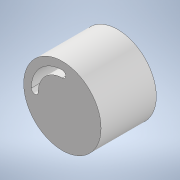
# Autodesk Inventor part: HandleGear2
Saved by Autodesk Inventor 2021 (Build 250183000, 183)
## iProperties
Created: 2021-03-29
Part Number: HandleGear2
Material: Generic
Document SubType Name: Modeling
Designer: ben
Density: 1 g/cm^3
Appearance: Default
Author: ben
Autodesk Inventor part; units mm, degrees
ref_plane "YZ Plane" through (0, 0, 0) normal (1, 0, 0) x (0, 1, 0)
ref_plane "XZ Plane" through (0, 0, 0) normal (0, 1, 0) x (-1, 0, 0)
ref_plane "XY Plane" through (0, 0, 0) normal (0, 0, 1) x (1, 0, 0)
sketch "Sketch1" plane through (0, 0, 0) normal (0, 0, 1) x (1, 0, 0)
  circle A0 centre (0.6539, 4.9671) radius 28 projected
  arc A1 (0.5947, 27.4671) -> (-21.846, 4.9079) centre (0.6539, 4.9671) ccw projected
  arc A2 (0.6079, 22.4671) -> (0.5947, 27.4671) centre (0.6013, 24.9671) ccw projected
  arc A3 (0.6079, 22.4671) -> (-16.846, 4.9211) centre (0.6539, 4.9671) ccw projected
  arc A4 (-21.846, 4.9079) -> (-16.846, 4.9211) centre (-19.346, 4.9145) ccw projected
  arc A5 (-3.34, -17.6834) -> (23.3045, 8.961) centre (0.6539, 4.9671) ccw
  line L0 (0.6539, 4.9671) -> (-3.34, -17.6834) construction
  line L1 (0.6539, 4.9671) -> (23.6539, 4.9671) construction
  line L2 (0.6539, 4.9671) -> (23.3045, 8.961) construction
  line L3 (-3.34, -17.6834) -> (-4.2082, -22.6075)
  line L4 (23.3045, 8.961) -> (28.2286, 9.8293)
  line L5 (-2.354, 4.7534) -> (-2.3232, 4.7704) projected
  line L6 (-2.3232, 4.7704) -> (3.4789, 4.0066) projected
  line L7 (3.4789, 4.0066) -> (3.5043, 3.9821) projected
  arc A6 (3.5043, 3.9821) -> (3.6402, 5.0151) centre (0.6431, 4.8842) ccw projected
  line L8 (3.6402, 5.0151) -> (3.6094, 4.998) projected
  line L9 (3.6094, 4.998) -> (-2.1927, 5.7619) projected
  line L10 (-2.1927, 5.7619) -> (-2.2181, 5.7864) projected
  arc A7 (-2.2181, 5.7864) -> (-2.354, 4.7534) centre (0.6431, 4.8842) ccw projected
  line L11 (3.4147, 6.0323) -> (2.8398, 5.3712) projected
  line L12 (2.8398, 5.3712) -> (3.6402, 5.0151) projected
  arc A8 (3.6402, 5.0151) -> (3.4147, 6.0323) centre (0.6431, 4.8842) ccw projected
  line L13 (2.8549, 6.911) -> (2.5407, 6.0932) projected
  line L14 (2.5407, 6.0932) -> (3.4147, 6.0323) projected
  arc A9 (3.4147, 6.0323) -> (2.8549, 6.911) centre (0.6431, 4.8842) ccw projected
  line L15 (2.0283, 7.5453) -> (2.0128, 6.6693) projected
  line L16 (2.0128, 6.6693) -> (2.8549, 6.911) projected
  arc A10 (2.8549, 6.911) -> (2.0283, 7.5453) centre (0.6431, 4.8842) ccw projected
  line L17 (2.0283, 7.5453) -> (2.0128, 6.6693) projected
  line L18 (2.0128, 6.6693) -> (2.8549, 6.911) projected
  arc A11 (2.8549, 6.911) -> (2.0283, 7.5453) centre (0.6431, 4.8842) ccw projected
  line L19 (1.3197, 7.0301) -> (2.0283, 7.5453) projected
  arc A12 (2.0283, 7.5453) -> (1.0347, 7.8586) centre (0.6431, 4.8842) ccw projected
  line L20 (1.0347, 7.8586) -> (1.3197, 7.0301) projected
  line L21 (0.545, 7.1321) -> (1.0347, 7.8586) projected
  arc A13 (1.0347, 7.8586) -> (-0.0062, 7.8131) centre (0.6431, 4.8842) ccw projected
  line L22 (-0.0062, 7.8131) -> (0.545, 7.1321) projected
  line L23 (-0.2179, 6.963) -> (-0.0062, 7.8131) projected
  arc A14 (-0.0062, 7.8131) -> (-0.9688, 7.4144) centre (0.6431, 4.8842) ccw projected
  line L24 (-0.9688, 7.4144) -> (-0.2179, 6.963) projected
  line L25 (-0.877, 6.5431) -> (-0.9688, 7.4144) projected
  arc A15 (-0.9688, 7.4144) -> (-1.737, 6.7105) centre (0.6431, 4.8842) ccw projected
  line L26 (-1.737, 6.7105) -> (-0.877, 6.5431) projected
  line L27 (-2.2181, 5.7864) -> (-1.3527, 5.9232) projected
  line L28 (-1.3527, 5.9232) -> (-1.737, 6.7105) projected
  arc A16 (-1.737, 6.7105) -> (-2.2181, 5.7864) centre (0.6431, 4.8842) ccw projected
  line L29 (-2.1285, 3.7362) -> (-1.5536, 4.3972) projected
  line L30 (-1.5536, 4.3972) -> (-2.354, 4.7534) projected
  arc A17 (-2.354, 4.7534) -> (-2.1285, 3.7362) centre (0.6431, 4.8842) ccw projected
  line L31 (-1.2545, 3.6753) -> (-2.1285, 3.7362) projected
  arc A18 (-2.1285, 3.7362) -> (-1.5687, 2.8575) centre (0.6431, 4.8842) ccw projected
  line L32 (-1.5687, 2.8575) -> (-1.2545, 3.6753) projected
  line L33 (-0.7266, 3.0992) -> (-1.5687, 2.8575) projected
  arc A19 (-1.5687, 2.8575) -> (-0.7421, 2.2232) centre (0.6431, 4.8842) ccw projected
  line L34 (-0.7421, 2.2232) -> (-0.7266, 3.0992) projected
  line L35 (-0.0335, 2.7384) -> (-0.7421, 2.2232) projected
  arc A20 (-0.7421, 2.2232) -> (0.2515, 1.9099) centre (0.6431, 4.8842) ccw projected
  line L36 (0.2515, 1.9099) -> (-0.0335, 2.7384) projected
  line L37 (0.7412, 2.6364) -> (0.2515, 1.9099) projected
  arc A21 (0.2515, 1.9099) -> (1.2924, 1.9553) centre (0.6431, 4.8842) ccw projected
  line L38 (1.2924, 1.9553) -> (0.7412, 2.6364) projected
  line L39 (1.5041, 2.8055) -> (1.2924, 1.9553) projected
  arc A22 (1.2924, 1.9553) -> (2.255, 2.3541) centre (0.6431, 4.8842) ccw projected
  line L40 (2.255, 2.3541) -> (1.5041, 2.8055) projected
  line L41 (3.0232, 3.058) -> (2.1632, 3.2254) projected
  line L42 (2.1632, 3.2254) -> (2.255, 2.3541) projected
  arc A23 (2.255, 2.3541) -> (3.0232, 3.058) centre (0.6431, 4.8842) ccw projected
  line L43 (3.5043, 3.9821) -> (2.6389, 3.8453) projected
  line L44 (2.6389, 3.8453) -> (3.0232, 3.058) projected
  arc A24 (3.0232, 3.058) -> (3.5043, 3.9821) centre (0.6431, 4.8842) ccw projected
  line L45 (0.6431, 4.8842) -> (-27.3459, 4.8842)
  line L46 (-29.3459, 4.8842) -> (-26.3459, 6.6163)
  line L47 (-26.3459, 6.6163) -> (-26.3459, 3.1522)
  line L48 (-26.3459, 3.1522) -> (-29.3459, 4.8842)
  point P0 (0, 0)
  point P1 (-27.318, 3.7134)
  point P2 (-27.3251, 6.051)
  dimension "d8" = 23
  dimension "d9" = 100
  dimension "d10" = 110
  dimension "d11" = 4.924
  dimension "d12" = 4.924
  dimension "d18" = 3
  constraints: 18 end point, 5 point on circle, 2 horizontal, 1 centre point, 1 coincident, 1 equal length, 1 point on line, 7 other
  measures "d8" radius of A5
  measures "d9" angle of L0 L1
  measures "d10" angle of L0 L2
  measures "d11" horizontal distance of L2.end L4.end
  measures "d12" vertical distance of L0.end L3.end
  measures "d18" horizontal distance of L46.start L46.end
ref_plane "Work Plane1" through (-27.427, -23.1101, -9.6285) normal (0, 0, 1) x (0.9999965, 0.0026331, 0)
extrude "Extrusion3" add sketch "Sketch1" along normal blind 35 contours L4 A5 L3 A0 L48 L47 L46 | L46 L47 L45 A0 | A0 L48 L46 | A0 L45 L47 L48 | A7 L10 L9 L8 A6 L7 L6 L5 | L30 L29 A17 | L31 L32 A18 | A16 L28 L27 | L33 L34 A19 | A24 L44 L43 | A15 L25 L26 | L35 L36 A20 | L12 L11 A8 | A23 L42 L41 | A14 L23 L24 | L37 L38 A21 | L14 L13 A9 | A22 L39 L40 | A13 L21 L22 | L16 L15 A10 | A12 L19 L20
sketch "Sketch3" plane through (0, 0, 35) normal (0, 0, 1) x (1, 0, 0)
  line L0 (23.3045, 8.961) -> (28.2286, 9.8293) projected
  arc A0 (28.2286, 9.8293) -> (-27.3251, 6.051) centre (0.6539, 4.9671) ccw projected
  line L1 (-27.3251, 6.051) -> (-29.3459, 4.8842) projected
  line L2 (-29.3459, 4.8842) -> (-27.318, 3.7134) projected
  arc A1 (-27.318, 3.7134) -> (-4.2082, -22.6075) centre (0.6539, 4.9671) ccw projected
  line L3 (-4.2082, -22.6075) -> (-3.34, -17.6834) projected
  arc A2 (-3.34, -17.6834) -> (23.3045, 8.961) centre (0.6539, 4.9671) ccw projected
  arc A3 (0.6079, 22.4671) -> (-16.846, 4.9211) centre (0.6539, 4.9671) ccw projected
  arc A4 (-21.846, 4.9079) -> (-16.846, 4.9211) centre (-19.346, 4.9145) ccw projected
  arc A5 (0.5947, 27.4671) -> (-21.846, 4.9079) centre (0.6539, 4.9671) ccw projected
  arc A6 (0.6079, 22.4671) -> (0.5947, 27.4671) centre (0.6013, 24.9671) ccw projected
  line L4 (3.6402, 5.0151) -> (3.6094, 4.998) projected
  line L5 (3.6094, 4.998) -> (-2.1927, 5.7619) projected
  line L6 (-2.1927, 5.7619) -> (-2.2181, 5.7864) projected
  line L7 (-2.2181, 5.7864) -> (-1.3527, 5.9232) projected
  line L8 (-1.3527, 5.9232) -> (-1.737, 6.7105) projected
  line L9 (-1.737, 6.7105) -> (-0.877, 6.5431) projected
  line L10 (-0.877, 6.5431) -> (-0.9688, 7.4144) projected
  line L11 (-0.9688, 7.4144) -> (-0.2179, 6.963) projected
  line L12 (-0.2179, 6.963) -> (-0.0062, 7.8131) projected
  line L13 (-0.0062, 7.8131) -> (0.545, 7.1321) projected
  line L14 (0.545, 7.1321) -> (1.0347, 7.8586) projected
  line L15 (1.0347, 7.8586) -> (1.3197, 7.0301) projected
  line L16 (1.3197, 7.0301) -> (2.0283, 7.5453) projected
  line L17 (2.0283, 7.5453) -> (2.0128, 6.6693) projected
  line L18 (2.0128, 6.6693) -> (2.8549, 6.911) projected
  line L19 (2.8549, 6.911) -> (2.5407, 6.0932) projected
  line L20 (2.5407, 6.0932) -> (3.4147, 6.0323) projected
  line L21 (3.4147, 6.0323) -> (2.8398, 5.3712) projected
  line L22 (2.8398, 5.3712) -> (3.6402, 5.0151) projected
  line L23 (-2.1285, 3.7362) -> (-1.5536, 4.3972) projected
  line L24 (-1.5536, 4.3972) -> (-2.354, 4.7534) projected
  line L25 (-2.354, 4.7534) -> (-2.3232, 4.7704) projected
  line L26 (-2.3232, 4.7704) -> (3.4789, 4.0066) projected
  line L27 (3.4789, 4.0066) -> (3.5043, 3.9821) projected
  line L28 (3.5043, 3.9821) -> (2.6389, 3.8453) projected
  line L29 (2.6389, 3.8453) -> (3.0232, 3.058) projected
  line L30 (3.0232, 3.058) -> (2.1632, 3.2254) projected
  line L31 (2.1632, 3.2254) -> (2.255, 2.3541) projected
  line L32 (2.255, 2.3541) -> (1.5041, 2.8055) projected
  line L33 (1.5041, 2.8055) -> (1.2924, 1.9553) projected
  line L34 (1.2924, 1.9553) -> (0.7412, 2.6364) projected
  line L35 (0.7412, 2.6364) -> (0.2515, 1.9099) projected
  line L36 (0.2515, 1.9099) -> (-0.0335, 2.7384) projected
  line L37 (-0.0335, 2.7384) -> (-0.7421, 2.2232) projected
  line L38 (-0.7421, 2.2232) -> (-0.7266, 3.0992) projected
  line L39 (-0.7266, 3.0992) -> (-1.5687, 2.8575) projected
  line L40 (-1.5687, 2.8575) -> (-1.2545, 3.6753) projected
  line L41 (-1.2545, 3.6753) -> (-2.1285, 3.7362) projected
  circle A7 centre (0.6539, 4.9671) radius 30
  point P0 (0, 0)
  dimension "d19" = 60
  constraints: 1 centre point, 1 coincident
  measures "d19" diameter of A7
extrude "Extrusion4" add sketch "Sketch3" against normal blind 5 contours A2 L3 A1 L2 L1 A0 L0 | A7 | A3 A4 A5 A6
sketch "Sketch4" plane through (0.6539, 4.9671, 35) normal (0, 0, 1) x (1, 0, 0)
  line L0 (0, 13.8567) -> (12.0002, -6.9283)
  line L1 (12.0002, -6.9283) -> (-12.0002, -6.9283)
  line L2 (-12.0002, -6.9283) -> (0, 13.8567)
  point P0 (-0.6539, -4.9671)
  point P1 (0, 0)
  point P2 (0, 0)
  dimension "d23" = 20.785
  constraints: 6 end point, 1 coincident, 7 other
  measures "d23" vertical distance of L0.start L0.end
extrude "Extrusion5" cut sketch "Sketch4" against normal blind 15
equation "\"BendRadius\" = Thickness"
equation "\"BendReliefWidth\" = Thickness"
equation "\"BendReliefDepth\" = 0.5 * Thickness"
equation "\"CornerReliefSize\" = 4 * Thickness"
equation "\"MinimumRemnant\" = 2 * Thickness"
equation "\"TransitionRadius\" = BendRadius"
equation "\"JacobiRadiusSize\" = Thickness"
equation "\"GapSize\" = Thickness"
equation "\"Thickness\" = 0.5"
body "Solid3"
